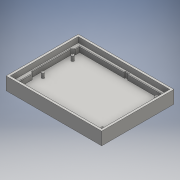
# Autodesk Inventor part: Lådaprototyp
Saved by Autodesk Inventor 2016 (Build 200138000, 138)
## iProperties
Created: 2018-02-27
Part Number: Lådaprototyp
Material: Generic
Document SubType Name: Modeling
Designer: Simon
Density: 1 g/cm^3
Appearance: Default
Author: Simon
Autodesk Inventor part; units mm, degrees
ref_plane "YZ Plane" through (0, 0, 0) normal (1, 0, 0) x (0, 1, 0)
ref_plane "XZ Plane" through (0, 0, 0) normal (0, 1, 0) x (-1, 0, 0)
ref_plane "XY Plane" through (0, 0, 0) normal (0, 0, 1) x (1, 0, 0)
sketch "Sketch1" plane through (0, 0, 0) normal (0, 0, 1) x (1, 0, 0)
  line L0 (0, 0) -> (90, 0)
  line L1 (90, 0) -> (90, 68)
  line L2 (90, 68) -> (0, 68)
  line L3 (0, 68) -> (0, 0)
  dimension "d0" = 90
  dimension "d1" = 68
  constraints: 8 end point, 2 parallel, 1 horizontal, 1 perpendicular
  measures "d0" distance of L2.end L1.end
  measures "d1" distance of L1.end L0.end
extrude "Extrusion1" add sketch "Sketch1" along normal blind 2
sketch "Sketch2" plane through (0, 0, 2) normal (0, 0, 1) x (1, 0, 0)
  line L0 (90, 68) -> (0, 68) projected
  line L1 (0, 68) -> (90, 68)
  line L2 (90, 68) -> (90, 0)
  line L3 (90, 0) -> (0, 0)
  line L4 (0, 0) -> (0, 68)
  line L5 (2, 66) -> (88, 66)
  line L6 (88, 66) -> (88, 2)
  line L7 (88, 2) -> (2, 2)
  line L8 (2, 2) -> (2, 66)
  dimension "d4" = 2
  dimension "d5" = 2
  dimension "d6" = 2
  dimension "d7" = 2
  constraints: 16 end point, 4 parallel, 2 horizontal, 2 perpendicular, 2 point on line
  measures "d4" distance between parallel lines of L7 L3
  measures "d5" distance between parallel lines of L0 L5
  measures "d6" distance between parallel lines of L6 L2
  measures "d7" distance between parallel lines of L4 L8
extrude "Extrusion2" add sketch "Sketch2" along normal blind 10
sketch "Sketch3" plane through (0, 0, 2) normal (0, 0, 1) x (1, 0, 0)
  line L0 (6, 63.2) -> (86, 63.2)
  line L1 (86, 63.2) -> (86, 4.8)
  line L2 (86, 4.8) -> (6, 4.8)
  line L3 (4, 21.3) -> (4, 57.2)
  line L4 (2, 66) -> (88, 66) projected
  line L5 (0, 0) -> (90, 0) projected
  line L6 (90, 68) -> (0, 68) projected
  line L7 (88, 2) -> (2, 2) projected
  line L8 (2, 2) -> (2, 66) projected
  line L9 (88, 66) -> (88, 2) projected
  line L10 (47.8, 63.2) -> (50.703, 63.2)
  line L11 (50.703, 63.2) -> (50.703, 64.6)
  line L12 (50.703, 64.6) -> (47.8, 64.6)
  line L13 (47.8, 64.6) -> (47.8, 63.2)
  circle A0 centre (82, 59.7) radius 1.5
  line L14 (4, 57.2) -> (6, 59.2)
  line L15 (4, 57.2) -> (6.8284, 57.2) construction
  line L16 (6, 59.2) -> (6, 63.2)
  line L17 (4, 21.3) -> (6, 19.3)
  line L18 (4, 21.3) -> (6.8284, 21.3) construction
  line L19 (6, 19.3) -> (6, 4.8)
  circle A1 centre (8.75, 53.95) radius 1.25
  circle A2 centre (8.75, 25.95) radius 1.25
  line L20 (86.5, 63.7) -> (5.5, 63.7)
  line L21 (5.5, 63.7) -> (5.5, 59.4071)
  line L22 (5.5, 59.4071) -> (3.5, 57.4071)
  line L23 (3.5, 57.4071) -> (3.5, 21.0929)
  line L24 (3.5, 21.0929) -> (5.5, 19.0929)
  line L25 (5.5, 19.0929) -> (5.5, 4.3)
  line L26 (5.5, 4.3) -> (86.5, 4.3)
  line L27 (86.5, 4.3) -> (86.5, 63.7)
  circle A3 centre (82, 8.8) radius 1.5
  dimension "d11" = 58.4
  dimension "d12" = 2.8
  dimension "d14" = 64
  dimension "d18" = 2
  dimension "d19" = 86
  dimension "d20" = 38.2
  dimension "d21" = 1.4
  dimension "d22" = 3
  dimension "d23" = 3.5
  dimension "d24" = 4
  dimension "d25" = 45
  dimension "d26" = 4
  dimension "d28" = 45
  dimension "d30" = 2
  dimension "d31" = 2
  dimension "d32" = 82
  dimension "d33" = 2.5
  dimension "d34" = 4.75
  dimension "d36" = 2.5
  dimension "d38" = 25.5
  dimension "d39" = 8
  dimension "d40" = 14.5
  dimension "d41" = 39.9
  dimension "d42" = 0.5
  dimension "d45" = 3
  dimension "d47" = 2.5
  constraints: 44 end point, 7 perpendicular, 6 parallel, 4 centre point, 4 horizontal, 2 equal length, 2 vertical alignment, 1 point on line, 7 other
  measures "d11" distance of L0.end L1.end
  measures "d12" distance between parallel lines of L0 L4
  measures "d14" distance between parallel lines of L7 L4
  measures "d18" distance between parallel lines of L8 L3
  measures "d19" distance between parallel lines of L9 L8
  measures "d20" distance between parallel lines of L13 L1
  measures "d21" distance of L10.end L11.end
  measures "d22" diameter of A0
  measures "d23" distance from line of L0 A0.centre
  measures "d24" distance from line of L1 A0.centre
  measures "d25" angle of L15 L14
  measures "d26" distance of L0.start L14.end
  measures "d28" angle of L17 L18
  measures "d30" distance between parallel lines of L3 L16
  measures "d31" distance between parallel lines of L3 L19
  measures "d32" distance between parallel lines of L1 L3
  measures "d33" diameter of A1
  measures "d34" distance from line of L3 A1.centre
  measures "d36" diameter of A2
  measures "d39" distance edge to line of A1 L0
  measures "d40" distance from line of L2 L17.end
  measures "d41" distance of L17.end L14.end
  measures "d42" distance between parallel lines of L0 L20
  measures "d45" diameter of A3
  measures "d47" distance edge to line of A3 L2
extrude "Extrusion3" add sketch "Sketch3" along normal blind 5
fillet "Fillet1" radius 1 4 edges at (7.5, 53.95, 7) (7.5, 25.95, 7) (80.5, 59.7, 7) (80.5, 8.8, 7)
fillet "Fillet2" radius 0.5 12 edges at (26.65, 63.7, 7) (5.5, 61.5536, 7) (4.5, 58.4071, 7) (3.5, 39.25, 7) (4.5, 20.0929, 7) (5.5, 11.6964, 7) (46, 4.3, 7) (86.5, 34, 7) (68.6015, 63.7, 7) (49.2515, 64.6, 7) (50.703, 64.15, 7) (47.8, 64.15, 7)
equation "\"d12\" = -0.5 * d11 + 0.5 * d14"
equation "\"d18\" = -0.5 * d10 + 0.5 * d19"
equation "\"d10\" = 82"
body "Solid1"
